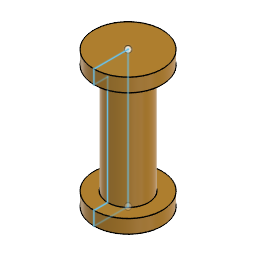
Simple gripper_Pin (Autodesk Fusion 360 design; units mm, degrees)
Autodesk Fusion 360 part; units mm, degrees
sketch "sketch 570" plane through (0, 0, 0) normal (1, 0, 0) x (0, 1, 0)
  line L0 (-94, 12) -> (-95, 12)
  line L1 (-94, 4) -> (-94, 12)
  line L2 (-95, 4) -> (-94, 4)
  line L3 (-95, 3) -> (-95, 4)
  line L4 (-92.5, 3) -> (-95, 3)
  line L5 (-92.5, 13) -> (-92.5, 3)
  line L6 (-95, 13) -> (-92.5, 13)
  line L7 (-95, 12) -> (-95, 13)
revolve "Revolve1" add sketch "sketch 570" angle 360 about axis through (0, -92.5, 13) along (0, 0, -1)
